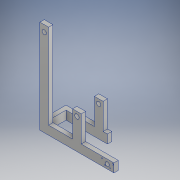
# Autodesk Inventor part: shooter
Saved by Autodesk Inventor 2019 (Build 230136000, 136)
## iProperties
Created: 2019-04-02
Part Number: shooter
Material: Aluminum 6061
Document SubType Name: Modeling
Designer: User
Density: 2.7 g/cm^3
Appearance: Aluminum - Flat
Mass: 367.89 g
Surface Area: 375.999 cm^2
Volume: 136.256 cm^3
Author: User
Autodesk Inventor part; units mm, degrees
ref_plane "YZ Plane" through (0, 0, 0) normal (1, 0, 0) x (0, 1, 0)
ref_plane "XZ Plane" through (0, 0, 0) normal (0, 1, 0) x (-1, 0, 0)
sketch "Sketch1" plane through (0, 0, 0) normal (1, 0, 0) x (0, 1, 0)
  line L0 (0, 0) -> (-228.6, 0)
  line L1 (-228.6, 0) -> (-228.6, -12.7)
  line L2 (-228.6, -12.7) -> (0, -12.7)
  line L3 (0, -12.7) -> (0, 0)
  line L4 (0, -12.7) -> (-88.9, -12.7)
  line L5 (-88.9, -63.5) -> (0, -63.5)
  line L6 (0, -63.5) -> (-228.6, -63.5)
  line L7 (-228.6, -63.5) -> (-228.6, -76.2)
  line L8 (-228.6, -76.2) -> (0, -76.2)
  line L9 (0, -76.2) -> (0, -63.5)
  line L10 (-228.6, 0) -> (-215.9, 0)
  line L11 (-215.9, 0) -> (-215.9, -76.2)
  line L12 (-215.9, -76.2) -> (-228.6, -76.2)
  line L13 (-228.6, -76.2) -> (-228.6, 0)
  dimension "d1" = 12.7
  dimension "d4" = 12.7
  dimension "d63" = 12.7
  dimension "d64" = 228.6
  dimension "d65" = 228.6
  dimension "d66" = 50.8
  constraints: 28 end point, 7 parallel, 4 horizontal, 3 perpendicular, 1 collinear, 1 point on line
  measures "d1" distance of L1.end L0.end
  measures "d4" distance of L6.end L7.end
  measures "d63" distance between parallel lines of L13 L11
  measures "d64" distance between parallel lines of L3 L1
  measures "d65" distance between parallel lines of L13 L9
  measures "d66" distance between parallel lines of L6 L2
extrude "Extrusion1" add sketch "Sketch1" along normal blind 25.4
sketch "Sketch3" plane through (0, -228.6, -76.2) normal (0, 0, -1) x (-1, 0, 0)
  line L0 (0, 0) -> (0, 228.6) projected
  line L1 (0, 228.6) -> (-25.4, 228.6) projected
  line L2 (-25.4, 0) -> (-25.4, 228.6) projected
  line L3 (0, 0) -> (-25.4, 0) projected
  point P0 (0, 228.6)
  point P1 (-12.7, 31.75)
  dimension "d18" = 25.4
  dimension "d19" = 12.7
  dimension "d20" = 31.75
  measures "d18" distance of L0.start L2.start
  measures "d19" distance from line of L2 point (-12.7, 31.75)
  measures "d20" distance from line of L3 point (-12.7, 31.75)
hole "Hole2" at (12.7, -196.85, -76.2) direction (0, 0, 1) diameter 11.9888 end through all
sketch "Sketch5" plane through (25.4, 0, 0) normal (1, 0, 0) x (0, 0, -1)
  line L0 (0, 0) -> (12.7, 0)
  line L1 (12.7, 0) -> (12.7, -25.4)
  line L2 (12.7, -25.4) -> (0, -25.4)
  line L3 (0, -25.4) -> (0, 0)
  line L4 (0, 0) -> (0, -228.6) projected
  line L5 (12.7, 0) -> (0, 0) projected
  dimension "d39" = 12.7
  dimension "d67" = 25.4
  dimension "d68" = 0
  dimension "d69" = 0
  constraints: 8 end point, 2 parallel, 1 horizontal, 1 perpendicular
  measures "d39" distance of L1.end L2.end
  measures "d67" distance between parallel lines of L2 L0
  measures "d68" distance between parallel lines of L5 L0
  measures "d69" distance between parallel lines of L3 L4
extrude "Extrusion2" add sketch "Sketch5" along normal blind 247.65
sketch "Sketch9" plane through (25.4, 0, 0) normal (1, 0, 0) x (0, 0, -1)
  line L0 (12.7, -215.9) -> (12.7, -25.4) projected
  line L1 (0, -95.25) -> (12.7, -95.25)
  line L2 (12.7, -95.25) -> (12.7, -120.65)
  line L3 (12.7, -120.65) -> (0, -120.65)
  line L4 (0, -120.65) -> (0, -95.25)
  line L5 (0, -25.4) -> (0, -228.6) projected
  line L6 (0, -25.4) -> (12.7, -25.4) projected
  point P0 (0, 0)
  dimension "d81" = 25.4
  dimension "d83" = 12.7
  dimension "d84" = 12.7
  dimension "d85" = 69.85
  constraints: 8 end point, 2 parallel, 1 horizontal, 1 midpoint, 1 perpendicular
  measures "d81" distance between parallel lines of L3 L1
  measures "d83" distance between parallel lines of L0 L5
  measures "d84" distance between parallel lines of L0 L4
  measures "d85" distance between parallel lines of L1 L6
extrude "Extrusion3" add sketch "Sketch9" along normal blind 76.2 contours L3 L4 L1 L0
sketch "Sketch8" plane through (0, -215.9, -12.7) normal (0, 0, -1) x (-1, 0, 0)
  line L0 (-273.05, 190.5) -> (-273.05, 215.9) projected
  line L1 (0, 215.9) -> (-273.05, 215.9) projected
  point P0 (-254, 203.2)
  dimension "d70" = 19.05
  dimension "d71" = 25.4
  dimension "d72" = 12.7
  measures "d70" distance from line of L0 point (-254, 203.2)
  measures "d71" distance of L0.start L0.end
  measures "d72" distance from line of L1 point (-254, 203.2)
hole "Hole6" at (254, -12.7, -12.7) direction (0, 0, 1) diameter 12.7 end through all
ref_plane "Work Plane1" through (0, -215.9, -38.1) normal (0, 0, 1) x (1, 0, 0)
mirror "Mirror1" about plane through (0, -215.9, -38.1) normal (0, 0, 1) of "Extrusion3"
sketch "Sketch10" plane through (0, -228.6, 0) normal (0, 0, 1) x (1, 0, 0)
  line L0 (25.4, 133.35) -> (101.6, 133.35) projected
  line L1 (25.4, 107.95) -> (101.6, 107.95) projected
  line L2 (101.6, 133.35) -> (101.6, 107.95) projected
  point P0 (0, 228.6)
  point P1 (88.9, 120.65)
  dimension "d89" = 25.4
  dimension "d90" = 12.7
  dimension "d91" = 12.7
  measures "d89" distance between parallel lines of L1 L0
  measures "d90" distance from line of L0 point (88.9, 120.65)
  measures "d91" distance from line of L2 point (88.9, 120.65)
hole "Hole7" at (88.9, -107.95, 0) direction (0, 0, -1) diameter 12.827 end through all
sketch "Sketch11" plane through (0, -215.9, -63.5) normal (0, 0, 1) x (1, 0, 0)
  line L0 (0, 215.9) -> (25.4, 215.9) projected
  line L1 (25.4, 215.9) -> (25.4, 120.65) projected
  line L2 (0, 215.9) -> (25.4, 215.9)
  line L3 (25.4, 215.9) -> (25.4, 203.2)
  line L4 (25.4, 203.2) -> (0, 203.2)
  line L5 (0, 203.2) -> (0, 215.9)
  dimension "d99" = 12.7
  constraints: 8 end point, 2 parallel, 1 horizontal, 1 perpendicular, 1 point on line
  measures "d99" distance between parallel lines of L0 L4
extrude "Extrusion4" add sketch "Sketch11" along normal up to surface (50.8 mm away)
sketch "Sketch12" plane through (25.4, 0, 0) normal (1, 0, 0) x (0, 0, -1)
  line L0 (76.2, -228.6) -> (76.2, 0) projected
  line L1 (76.2, -133.35) -> (63.5, -133.35)
  line L2 (63.5, -12.7) -> (63.5, -215.9) projected
  line L3 (76.2, -120.65) -> (63.5, -120.65) projected
  line L4 (12.7, -215.9) -> (12.7, -12.7) projected
  line L5 (0, 0) -> (0, -228.6) projected
  line L6 (76.2, -120.65) -> (63.5, -120.65) projected
  line L7 (63.5, -120.65) -> (63.5, -215.9) projected
  line L8 (63.5, -215.9) -> (12.7, -215.9) projected
  line L9 (12.7, -215.9) -> (12.7, -120.65) projected
  line L10 (12.7, -120.65) -> (0, -120.65) projected
  line L11 (0, -120.65) -> (0, -228.6) projected
  line L12 (0, -228.6) -> (76.2, -228.6) projected
  line L13 (76.2, -228.6) -> (76.2, -120.65) projected
  line L14 (12.7, -215.9) -> (0, -215.9)
  dimension "d102" = 12.7
  constraints: 4 end point, 3 point on line, 1 horizontal, 1 perpendicular
  measures "d102" distance between parallel lines of L3 L1
extrude "Extrusion5" cut sketch "Sketch12" against normal blind 50.8 contours L12 L5 L14 L8 L2 L1 L0
sketch "Sketch13" plane through (0, 0, 0) normal (0, 0, 1) x (1, 0, 0)
  circle A0 centre (12.7, -196.85) radius 5.9944 projected
  point P0 (0, 0)
  point P1 (6.2738, -189.103)
  point P2 (19.7104, -181.356)
  point P3 (19.7104, -212.344)
  point P4 (6.2738, -204.597)
  dimension "d105" = 7.747
  dimension "d106" = 6.4262
  dimension "d107" = 7.0104
  dimension "d108" = 15.494
  dimension "d109" = 15.494
  dimension "d110" = 7.0104
  dimension "d111" = 7.747
  dimension "d112" = 6.4262
  measures "d105" vertical distance of point (6.274, -189.103) A0.centre
  measures "d106" horizontal distance of A0.centre point (6.274, -189.103)
  measures "d107" horizontal distance of A0.centre point (19.71, -181.356)
  measures "d108" vertical distance of A0.centre point (19.71, -181.356)
  measures "d109" vertical distance of A0.centre point (19.71, -212.344)
  measures "d110" horizontal distance of A0.centre point (19.71, -212.344)
  measures "d111" vertical distance of point (6.274, -204.597) A0.centre
  measures "d112" horizontal distance of A0.centre point (6.274, -204.597)
hole "Hole8" at (6.2738, -189.103, 0) at (19.7104, -181.356, 0) at (19.7104, -212.344, 0) at (6.2738, -204.597, 0) direction (0, 0, -1) diameter 3.175 end through all
equation "\"d4\" = d1"
equation "\"d65\" = d64"
equation "\"d19\" = 0.5 * d18"
equation "\"d84\" = d83"
equation "\"d72\" = 0.5 * d71"
equation "\"d90\" = 0.5 * d89"
equation "\"d109\" = d108"
equation "\"d110\" = d107"
equation "\"d111\" = d105"
equation "\"d112\" = d106"
body "Solid1"
